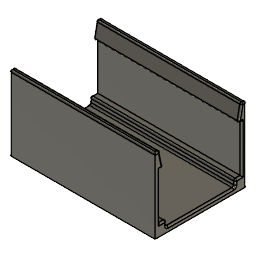
Prichytka_neon_LED_pasek_v1 (Autodesk Fusion 360 design; units mm, degrees)
Autodesk Fusion 360 part; units mm, degrees
sketch "Sketch1" plane through (0, 0, 0) normal (0, 0, 1) x (1, 0, 0)
  line L0 (9, -5.65) -> (-9, -5.65)
  line L1 (-9, -5.65) -> (-9, 5.65)
  line L2 (-9, 5.65) -> (9, 5.65)
  line L3 (9, 5.65) -> (9, -5.65)
  line L4 (9, -5.65) -> (-9, 5.65) construction
  line L5 (-9, -5.65) -> (9, 5.65) construction
  line L6 (-9, 4.25) -> (9, 4.25)
  line L7 (-9, -4.25) -> (9, -4.25)
  line L8 (-9, 5.05) -> (9, 5.05)
  line L9 (-9, -5.05) -> (9, -5.05)
  circle A0 centre (0, 0) radius 2
  dimension "d1" = 18
  dimension "d2" = 11.3
  dimension "d5" = 1.4
  dimension "d6" = 1.4
  dimension "d9" = 0.6
  dimension "d10" = 0.6
  dimension "d21" = 4
  constraint horizontal L0
  constraint perpendicular L0 L1
  constraint parallel L0 L2
  constraint parallel L1 L3
  constraint coincident L4 A0.centre
  constraint coincident L5 A0.centre
  constraint coincident A0.centre origin
  constraint coincident L1 L6.start
  constraint coincident L3 L6.end
  constraint perpendicular L3 L6
  constraint coincident L1 L7.start
  constraint coincident L3 L7.end
  constraint perpendicular L3 L7
  constraint coincident L1 L8.start
  constraint coincident L3 L8.end
  constraint perpendicular L3 L8
  constraint coincident L1 L9.start
  constraint coincident L3 L9.end
  constraint perpendicular L3 L9
  measures "d1" distance of L1.end L2.end
  measures "d2" distance of L0.end L1.end
  measures "d5" distance of L2 L6
  measures "d6" distance of L0 L7
  measures "d9" distance of L2 L8
  measures "d10" distance of L0 L9
  measures "d21" diameter of A0
extrude "Extrude1" add sketch "Sketch1" along normal blind 0.6
extrude "Extrude2" add sketch "Sketch1" along normal blind 1.4 contours L0 L1 L3 L9 | L1 L3 L7 L9 | L1 L3 L6 L8 | L1 L2 L3 L8
extrude "Extrude3" add sketch "Sketch1" along normal blind 9.2 contours L0 L1 L3 L9 | L1 L2 L3 L8
sketch "Sketch2" plane through (-9, 0, 0) normal (-1, 0, 0) x (0, -1, 0)
  line L0 (5.05, 1.4) -> (4.25, 1.4)
  line L1 (4.25, 1.4) -> (4.25, 0.6)
  line L2 (4.25, 0.6) -> (-4.25, 0.6)
  line L3 (-4.25, 0.6) -> (-4.25, 1.4)
  line L4 (-4.25, 1.4) -> (-5.05, 1.4)
  line L5 (-5.05, 1.4) -> (-5.05, 9.2)
  line L6 (-5.05, 9.2) -> (-5.65, 9.2)
  line L7 (-5.65, 9.2) -> (-5.65, 0)
  line L8 (-5.65, 0) -> (5.65, 0)
  line L9 (5.05, 9.2) -> (5.05, 1.4)
  line L10 (4.65, 7.2) -> (5.05, 7.2)
  line L11 (4.65, 7.2) -> (5.05, 9.2)
  line L12 (5.05, 7.2) -> (5.05, 9.2)
  line L13 (0, 0) -> (0, 9)
  line L14 (-4.65, 7.2) -> (-5.05, 9.2)
  line L15 (-5.05, 7.2) -> (-5.05, 9.2)
  line L16 (-4.65, 7.2) -> (-5.05, 7.2)
  point P0 (-5.05, 9.2)
  constraint coincident L9 L10.end
  constraint perpendicular L9 L10
  constraint coincident L9.start L11.end
  constraint coincident L13.start origin
  constraint perpendicular L8 L13
  constraint symmetric L9.start L13 P0
  constraint symmetric L10.start L13 L14.start
  constraint symmetric L10.end L13 L15.start
extrude "Extrude4" add sketch "Sketch2" against normal blind 18 contours L5 L14 L15 L16 | L9 L10 L11 L12
fillet "Fillet1" radius 0.2 39 edges at (0, 4.65, 7.2) (0, -4.65, 7.2) (0, -4.25, 1.4) (0, 4.25, 1.4) (0, 4.25, 0.6) (0, -4.25, 0.6) (-9, 5.65, 4.6) (-9, 4.85, 8.2) (-9, 5.05, 4.3) (-9, 4.85, 7.2) (-9, -4.85, 7.2) (-9, -5.05, 4.3) (-9, -4.85, 8.2) (9, -4.85, 8.2) (9, -4.85, 7.2) (9, -5.05, 4.3) (9, 5.05, 4.3) (9, 4.85, 8.2) (9, 4.85, 7.2) (9, -4.65, 1.4) (9, 4.65, 1.4) (9, 4.25, 1) (9, -4.25, 1) (9, 0, 0.6) (-9, 0, 0.6) (-9, 4.65, 1.4) (-9, 4.25, 1) (-9, -4.25, 1) (-9, -4.65, 1.4) (-9, -5.65, 4.6) (-9, -5.35, 9.2) (0, -5.65, 9.2) (0, 5.65, 9.2) (0, 5.05, 9.2) (-9, 5.35, 9.2) (9, 5.35, 9.2) (9, -5.35, 9.2) (0, -5.05, 9.2) (9, 5.65, 4.6)
chamfer "Chamfer1" distance 0.2 angle 45 1 edges at (-1.8647, 0.7232, 0.6)
